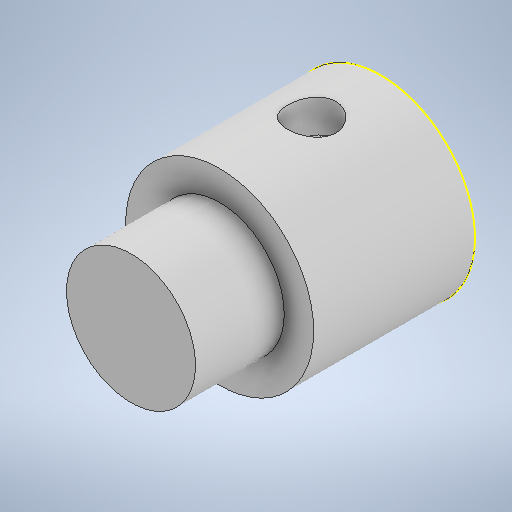
# Autodesk Inventor part: shaft_extension2
Saved by Autodesk Inventor 2025 (Build 290162000, 162)
## iProperties
Created: 2024-06-18
Part Number: shaft_extension2
Material: Generic
Document SubType Name: Modeling
Designer: Pintu
Density: 1 g/cm^3
Appearance: Default
Author: Pintu
Autodesk Inventor part; units mm, degrees
ref_plane "YZ Plane" through (0, 0, 0) normal (1, 0, 0) x (0, 1, 0)
ref_plane "XZ Plane" through (0, 0, 0) normal (0, 1, 0) x (-1, 0, 0)
sketch "Sketch1" plane through (0, 0, 0) normal (0, 0, 1) x (1, 0, 0)
  circle A0 centre (0, 0) radius 3.825
  circle A1 centre (0, 0) radius 5.825
  dimension "d0" = 7.65
  dimension "d1" = 2
  constraints: 2 centre point, 1 coincident
  measures "d0" diameter of A0
  measures "d1" radial gap between concentric circles of A0 A1
extrude "Extrusion1" add sketch "Sketch1" along normal blind 10
sketch "Sketch2" plane through (0, 0, 10) normal (0, 0, 1) x (1, 0, 0)
  circle A0 centre (0, 0) radius 4
  dimension "d4" = 8
  constraints: 1 centre point, 1 coincident
  measures "d4" diameter of A0
extrude "Extrusion2" add sketch "Sketch2" along normal mid plane 6
move faces "Move1" translate (0, 0, 2.5) faces at (0.7574, 1.0973, 13)
sketch "Sketch3" plane through (0, 0, 0) normal (0, 0, -1) x (-1, 0, 0)
  line L0 (0, 0) -> (0, 5.825)
  circle A0 centre (0, 0) radius 5.825 projected
  constraints: 2 end point, 1 vertical, 1 vertical alignment, 1 other
ref_plane "Work Plane1" through (0, 5.825, 0) normal (0, 1, 0) x (-1, 0, 0)
sketch "Sketch4" plane through (0, 5.825, 0) normal (0, 1, 0) x (-1, 0, 0)
  circle A0 centre (0, 4.3) radius 1.5
  point P0 (0, 0)
  dimension "d10" = 3
  dimension "d11" = 4.3
  constraints: 1 centre point
  measures "d10" diameter of A0
  measures "d11" distance of point (0, 0) A0.centre
extrude "Extrusion3" cut sketch "Sketch4" against normal through all
body "Solid1"
